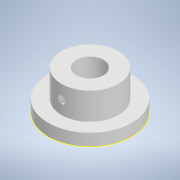
# Autodesk Inventor part: Деталь3
Saved by Autodesk Inventor 2022 (Build 260153000, 153)
## iProperties
Created: 2021-04-17
Part Number: Деталь3
Material: Типовые
Document SubType Name: Modeling
Designer: lbfas
Density: 1 g/cm^3
Appearance: По умолчанию
Author: lbfas
Autodesk Inventor part; units mm, degrees
ref_plane "YZ Plane" through (0, 0, 0) normal (1, 0, 0) x (0, 1, 0)
ref_plane "XZ Plane" through (0, 0, 0) normal (0, 1, 0) x (-1, 0, 0)
sketch "Эскиз1" plane through (0, 0, 0) normal (0, 1, 0) x (-1, 0, 0)
  circle A0 centre (0, 0) radius 9.5
  dimension "d0" = 19
  constraints: 1 centre point, 1 coincident
  measures "d0" diameter of A0
extrude "Выдавливание1" add sketch "Эскиз1" along normal blind 9
sketch "Эскиз2" plane through (0, 0, 0) normal (0, -1, 0) x (1, 0, 0)
  circle A0 centre (0, 0) radius 14
  constraints: 1 centre point
extrude "Выдавливание2" add sketch "Эскиз2" along normal blind 4
sketch "Эскиз3" plane through (0, 9, 0) normal (0, 1, 0) x (1, 0, 0)
  point P0 (0, 0)
hole "Отверстие1" at (0, 9, 0) direction (0, -1, 0) diameter 9 end through all
sketch "Эскиз4" plane through (0, -4, 0) normal (0, -1, 0) x (1, 0, 0)
  line L0 (0, 0) -> (0, 9)
  circle A0 centre (0, 9) radius 2.5
  circle A1 centre (-9, 0) radius 2.5
  circle A2 centre (0, -9) radius 2.5
  circle A3 centre (9, 0) radius 2.5
  dimension "d13" = 9
  dimension "d14" = 5
  dimension "d17" = 360
  constraints: 4 centre point, 2 end point, 1 coincident, 1 vertical, 9 other
  measures "d13" distance of L0.start L0.end
  measures "d14" diameter of A0
extrude "Выдавливание3" cut sketch "Эскиз4" against normal blind 2.5
sketch "Эскиз7" plane through (0, 0, 0) normal (0, 0, 1) x (1, 0, 0)
  circle A0 centre (0, 4.5) radius 1.25
  point P0 (0, 0)
  dimension "d37" = 2.5
  constraints: 1 centre point
  measures "d37" diameter of A0
sketch "Эскиз9" plane through (0, -4, 0) normal (0, -1, 0) x (1, 0, 0)
  circle A0 centre (-9, 0) radius 2.5 projected
  line L0 (-9, 2.5) -> (-3.7417, 2.5)
  circle A1 centre (0, 0) radius 4.5 projected
  line L1 (-9, -2.5) -> (-3.7417, -2.5)
  circle A2 centre (0, 9) radius 2.5 projected
  line L2 (-2.5, 9) -> (-2.5, 3.7417)
  line L3 (2.5, 9) -> (2.5, 3.7417)
  circle A3 centre (9, 0) radius 2.5 projected
  line L4 (9, 2.5) -> (3.7417, 2.5)
  line L5 (9, -2.5) -> (3.7417, -2.5)
  circle A4 centre (0, -9) radius 2.5 projected
  line L6 (2.5, -9) -> (2.5, -3.7417)
  line L7 (-2.5, -9) -> (-2.5, -3.7417)
  constraints: 16 end point, 6 point on line, 4 point on circle, 3 horizontal, 2 perpendicular, 2 tangent, 1 parallel, 13 other
extrude "Выдавливание4" cut sketch "Эскиз9" against normal blind 2.5 contours A0 L0 A1 L1 | L2 A2 L3 A1 | A1 L6 A4 L7 | L4 A3 L5 A1
fillet "Сопряжение3" radius 2.5 12 edges at (11.5, -1.5, 0) (6.3708, -1.5, -2.5) (6.3708, -1.5, 2.5) (2.5, -1.5, 6.3708) (-2.5, -1.5, 6.3708) (0, -1.5, 11.5) (-6.3708, -1.5, 2.5) (-6.3708, -1.5, -2.5) (-11.5, -1.5, 0) (0, -1.5, -11.5) (-2.5, -1.5, -6.3708) (2.5, -1.5, -6.3708)
extrude "Выдавливание5" cut sketch "Эскиз7" along normal blind 11.5
ref_plane "РабПлоскость1" through (0, 4.5, 0) normal (1, 0, 0) x (0, 0, 1)
sketch "Эскиз11" plane through (0, 4.5, 0) normal (1, 0, 0) x (0, 0, 1)
  line L0 (4.5, 1.25) -> (9.5, 1.25) projected
  line L1 (9.2113, 1.25) -> (9.2113, 1.75)
  line L2 (4.5, 6) -> (4.5, -4.5) projected
  line L3 (9.2113, 1.75) -> (8.9226, 1.25)
  line L4 (9.2113, 1.75) -> (9.5, 1.25)
  line L5 (8.9226, 1.25) -> (9.5, 1.25)
  point P0 (0, 4.5)
  dimension "d42" = 30
  dimension "d43" = 0.5
  dimension "d44" = 0.5774
  dimension "d45" = 0.5
  constraints: 8 end point, 1 horizontal, 1 symmetric about line
  measures "d42" angle of L3 L1
  measures "d43" vertical distance of L1.end L3.end
  measures "d44" distance of L3.end L4.end
  measures "d45" vertical distance of L1.end L4.end
coil "Пружина2" sketch "Эскиз11" operation cut axis through (0, 4.5, 0) along (0, 0, -1) pitch 0.577 turns 17.331023 hand right
sketch "Эскиз12" plane through (0, -4, 0) normal (0, -1, 0) x (1, 0, 0)
  circle A0 centre (0, 0) radius 14 projected
  line L0 (-14, 0) -> (14, 0)
  line L1 (0, -14) -> (0, 14)
  constraints: 4 end point, 4 point on circle, 1 horizontal, 1 perpendicular
